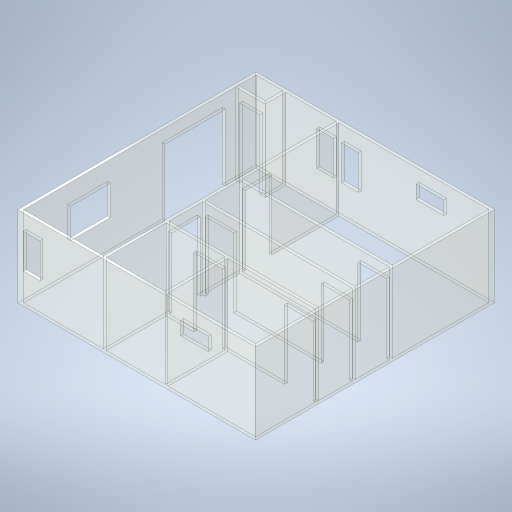
# Autodesk Inventor part: Interior_Walls
Saved by Autodesk Inventor 2024 (Build 280153000, 153)
## iProperties
Created: 2023-05-16
Part Number: Interior_Walls
Material: Steel
Document SubType Name: Modeling
Designer: Tom
Density: 7.85 g/cm^3
Appearance: Clear
Mass: 7.46669e+07 g
Surface Area: 2.27384e+06 cm^2
Volume: 9.51171e+06 cm^3
Author: Tom
Autodesk Inventor part; units mm, degrees
ref_plane "YZ Plane" through (0, 0, 0) normal (1, 0, 0) x (0, 1, 0)
ref_plane "XZ Plane" through (0, 0, 0) normal (0, 1, 0) x (-1, 0, 0)
ref_plane "XY Plane" through (0, 0, 0) normal (0, 0, 1) x (1, 0, 0)
sketch "Sketch1" plane through (0, 0, 0) normal (0, 1, 0) x (-1, 0, 0)
  line L0 (3606.8, -3606.8) -> (-3606.8, -3606.8)
  line L1 (-3606.8, -3606.8) -> (-3594.1, 3606.8)
  line L2 (-3594.1, 3606.8) -> (3594.1, 3606.8)
  line L3 (3594.1, 3606.8) -> (3606.8, -3606.8)
  line L4 (0, -3606.8) -> (0, 3606.8)
  line L5 (3600.45, 0) -> (-3600.45, 0)
  line L6 (3505.3564, 3517.9) -> (-3505.3564, 3517.9)
  line L7 (-3505.3564, 3517.9) -> (-3517.7433, -3517.9)
  line L8 (-3517.7433, -3517.9) -> (3517.7433, -3517.9)
  line L9 (3517.7433, -3517.9) -> (3505.3564, 3517.9)
  line L10 (-2204.4316, 514.35) -> (-2204.4316, 603.25)
  line L11 (5.3684, -603.25) -> (5.3684, -514.35)
  point P0 (0, 0)
  point P1 (0, 0)
  point P2 (-3511.5499, 0)
  dimension "d1" = 7213.6
  dimension "d2" = 12.7
  dimension "d4" = 7188.2
  dimension "d5" = 7213.6
  dimension "d6" = 88.9
  constraints: 24 end point, 6 midpoint, 2 parallel, 1 coincident, 1 horizontal, 1 perpendicular, 3 other
  measures "d1" distance of L0.start L0.end
  measures "d2" horizontal distance of L0.start L2.end
  measures "d4" distance of L1.end L2.end
  measures "d5" distance of L0.end L1.end
  measures "d6" distance between parallel lines of L2 L6
extrude "Extrusion1" add sketch "Sketch1" along normal blind 2438.4 contours L0 L4 L8 L9 L5 L3 | L0 L1 L5 L7 L8 L4 | L5 L9 L6 L4 L2 L3 | L1 L2 L4 L6 L7 L5
sketch "Sketch2" plane through (0, 2438.4, 0) normal (0, 1, 0) x (1, 0, 0)
  line L0 (-3517.7433, 3517.9) -> (3517.7433, 3517.9) projected
  line L1 (3505.3564, -3517.9) -> (-3505.3564, -3517.9) projected
  line L2 (-3517.7433, 3517.9) -> (3517.7433, 3517.9) projected
  line L3 (3505.3564, -3517.9) -> (-3505.3564, -3517.9) projected
  line L4 (3517.7433, 3517.9) -> (3505.3564, -3517.9) projected
  line L5 (-1009.4936, -1619.25) -> (3508.5426, -1619.25)
  line L6 (3508.5426, -1619.25) -> (3508.5426, -1708.15)
  line L7 (3508.5426, -1708.15) -> (-1009.4936, -1708.15)
  line L8 (857.4064, -1708.15) -> (768.5064, -1708.15)
  line L9 (768.5064, -1708.15) -> (768.5064, -3517.9)
  line L10 (768.5064, -3517.9) -> (857.4064, -3517.9)
  line L11 (857.4064, -3517.9) -> (857.4064, -1708.15)
  line L12 (-1009.4936, -3517.9) -> (-1009.4936, 3517.9)
  line L13 (-1098.3936, 3517.9) -> (-1098.3936, -3517.9)
  line L14 (-1009.4936, 3517.9) -> (-1098.3936, 3517.9)
  line L15 (-1009.4936, -3517.9) -> (-1098.3936, -3517.9)
  line L16 (-5.3684, -603.25) -> (2204.4316, -603.25) projected
  line L17 (-1009.4936, -603.25) -> (-1009.4936, -514.35)
  line L18 (-3505.3564, -3517.9) -> (-3517.7433, 3517.9) projected
  line L19 (-3516.6477, 2895.6) -> (-2614.9477, 2895.6)
  line L20 (-2703.8477, 2984.5) -> (-3516.6477, 2984.5)
  line L21 (-3516.6477, 2984.5) -> (-3516.6477, 2895.6)
  line L22 (-2703.8477, 2984.5) -> (-2703.8477, 3517.9)
  line L23 (-2703.8477, 3517.9) -> (-2614.9477, 3517.9)
  line L24 (-2614.9477, 3517.9) -> (-2614.9477, 2895.6)
  line L25 (-1009.4936, -603.25) -> (3510.6443, -603.25)
  line L26 (3510.6443, -603.25) -> (3510.6443, -514.35)
  line L27 (3510.6443, -514.35) -> (-1009.4936, -514.35)
  line L28 (-1009.4936, -514.35) -> (-1009.4936, -603.25)
  line L29 (-1009.4936, -1708.15) -> (-1009.4936, -1619.25)
  line L30 (-1009.4936, 514.35) -> (3512.6119, 514.35)
  line L31 (3512.6119, 514.35) -> (3512.6119, 603.25)
  line L32 (3512.6119, 603.25) -> (-1009.4936, 603.25)
  line L33 (-1009.4936, 603.25) -> (-1009.4936, 514.35)
  point P0 (0, 0)
  point P1 (857.4064, -3517.9)
  point P2 (768.5064, -1708.15)
  point P3 (-1098.3936, 3517.9)
  point P4 (-1098.3936, -3517.9)
  point P5 (-1009.4936, -3517.9)
  point P6 (-2614.9477, 3517.9)
  point P7 (-2703.8477, 3517.9)
  point P8 (-1009.4936, 603.25)
  dimension "d41" = 88.9
  dimension "d44" = 2647.95
  dimension "d45" = 1778
  dimension "d88" = 533.4
  dimension "d90" = 812.8
  dimension "d137" = 1016
  dimension "d138" = 514.35
  dimension "d139" = 514.35
  constraints: 54 end point, 16 point on line, 10 parallel, 9 perpendicular, 7 equal length, 5 horizontal, 2 collinear
  measures "d41" distance between parallel lines of L13 L12
  measures "d44" distance from line of L1.start L11
  measures "d45" distance between parallel lines of L9 L12
  measures "d88" distance of L20.start L22.end
  measures "d90" distance of L20.start L20.end
  measures "d137" distance between parallel lines of L5 L25
  measures "d138" distance from line of point (0, 0) L27
  measures "d139" distance from line of L30 point (0, 0)
extrude "Extrusion2" add sketch "Sketch2" against normal blind 2438.4 contours L0 L24 L19 L21 L20 L22 | L0 L12 L1 L13 | L32 L4 L30 L12 | L9 L7 L11 L1 | L12 L5 L6 L7 | L31 L30 L4 | L27 L4 L25 L16 L12 | L26 L25 L4
sketch "Sketch3" plane through (768.5064, 2438.4, 1708.15) normal (0, 0, 1) x (1, 0, 0)
  line L0 (-1778, -2438.4) -> (2740.0362, -2438.4) projected
  line L1 (2663.8362, -2438.4) -> (1800.2362, -2438.4)
  line L2 (1800.2362, -2438.4) -> (1800.2362, -355.6)
  line L3 (1800.2362, -355.6) -> (2663.8362, -355.6)
  line L4 (2663.8362, -355.6) -> (2663.8362, -2438.4)
  line L5 (2740.0362, 0) -> (2740.0362, -2438.4) projected
  point P0 (-768.5064, -2438.4)
  point P1 (-1526.4792, -2438.4)
  dimension "d36" = 76.2
  dimension "d37" = 863.6
  dimension "d38" = 2082.8
  constraints: 8 end point, 2 parallel, 1 horizontal, 1 perpendicular, 1 point on line
  measures "d36" distance between parallel lines of L5 L4
  measures "d37" distance of L2.end L3.end
  measures "d38" distance of L1.end L2.end
extrude "Extrusion3" cut sketch "Sketch3" against normal up to surface (2311.4 mm away)
ref_plane "Work Plane1" through (3038.6426, 2082.8, 1708.15) normal (0, -1, 0) x (1, 0, 0)
sketch "Sketch4" plane through (-0.1006, 2082.8, 57.15) normal (0, 1, 0) x (1, 0, 0)
  line L0 (857.507, -1651) -> (3508.6432, -1651) projected
  arc A0 (2594.2432, -1651) -> (3400.6932, -2457.45) centre (3400.6932, -1651) ccw
  line L1 (3400.6932, -1651) -> (2594.2432, -1651)
  line L2 (3400.6932, -1651) -> (3400.6932, -2457.45)
  point P0 (0.1006, 57.15)
  point P1 (3432.4432, -1651)
  dimension "d46" = 31.75
  dimension "d48" = 806.45
  constraints: 4 end point, 2 point on circle, 2 point on line, 1 centre point, 1 coincident, 1 perpendicular
  measures "d46" distance of point (3432.443, -1651) point (3400.693, -1651)
  measures "d48" distance of L1.start L1.end
sketch "Sketch5" plane through (-3594.1, 0, 3606.8) normal (0, 0, 1) x (1, 0, 0)
  line L0 (4927.6, 2006.6) -> (5753.1, 2006.6)
  line L1 (5753.1, 2006.6) -> (5753.1, 1600.2)
  line L2 (5753.1, 1600.2) -> (4927.6, 1600.2)
  line L3 (4927.6, 1600.2) -> (4927.6, 2006.6)
  line L4 (0, 0) -> (7188.2, 0) projected
  line L5 (7200.9, 0) -> (7200.9, 2438.4) projected
  point P0 (3594.1, 0)
  dimension "d51" = 2006.6
  dimension "d53" = 825.5
  dimension "d54" = 406.4
  dimension "d165" = 1447.8
  constraints: 8 end point, 2 parallel, 1 horizontal, 1 perpendicular
  measures "d51" distance between parallel lines of L4 L0
  measures "d53" distance of L0.start L0.end
  measures "d54" distance between parallel lines of L2 L0
  measures "d165" distance between parallel lines of L5 L1
extrude "Extrusion4" cut sketch "Sketch5" against normal up to surface (88.9 mm away)
sketch "Sketch6" plane through (3606.8, 0, -3606.8) normal (0, 0, -1) x (-1, 0, 0)
  line L0 (1447.8, 2006.6) -> (2286, 2006.6)
  line L1 (2286, 2006.6) -> (2286, 1600.2)
  line L2 (2286, 1600.2) -> (1447.8, 1600.2)
  line L3 (1447.8, 1600.2) -> (1447.8, 2006.6)
  line L4 (0, 0) -> (7213.6, 0) projected
  line L5 (0, 0) -> (0, 2438.4) projected
  point P0 (3606.8, 0)
  point P1 (1447.8, 1803.4)
  dimension "d57" = 2006.6
  dimension "d58" = 406.4
  dimension "d59" = 838.2
  dimension "d60" = 1447.8
  constraints: 8 end point, 2 parallel, 1 horizontal, 1 midpoint, 1 perpendicular
  measures "d57" distance between parallel lines of L4 L0
  measures "d58" distance of L2.end L0.start
  measures "d59" distance of L1.end L2.end
  measures "d60" distance from line of L5 point (1447.8, 1803.4)
extrude "Extrusion5" cut sketch "Sketch6" against normal up to surface (88.9 mm away)
sketch "Sketch7" plane through (-3517.7433, 0, -3517.9) normal (0.9999985, 0, -0.0017606) x (-0.0017606, 0, -0.9999985)
  line L0 (-927.1, 0) -> (-2755.9, 0)
  line L1 (-2755.9, 0) -> (-2755.9, 2006.6)
  line L2 (-2755.9, 2006.6) -> (-927.1, 2006.6)
  line L3 (-927.1, 2006.6) -> (-927.1, 0)
  line L4 (0, 0) -> (0, 2438.4) projected
  line L5 (-7035.8109, 0) -> (-622.301, 0) projected
  point P0 (-3524.0877, 0)
  dimension "d63" = 927.1
  dimension "d64" = 2006.6
  dimension "d65" = 1828.8
  constraints: 8 end point, 2 parallel, 1 collinear, 1 horizontal, 1 perpendicular
  measures "d63" distance between parallel lines of L3 L4
  measures "d64" distance of L0.end L1.end
  measures "d65" distance of L1.end L2.end
extrude "Extrusion6" cut sketch "Sketch7" against normal up to surface (88.9 mm away)
sketch "Sketch8" plane through (-3594.1, 0, 3606.8) normal (-0.9999985, 0, 0.0017606) x (0.0017606, 0, 0.9999985)
  line L0 (-2717.8, 1816.1) -> (-1511.3, 1816.1)
  line L1 (-1511.3, 1816.1) -> (-1511.3, 914.4)
  line L2 (-1511.3, 914.4) -> (-2717.8, 914.4)
  line L3 (-2717.8, 914.4) -> (-2717.8, 1816.1)
  line L4 (0, 0) -> (0, 2438.4) projected
  line L5 (-7213.6112, 0) -> (0, 0) projected
  point P0 (-3600.4668, 0)
  point P1 (-4368.6545, 0)
  dimension "d71" = 2717.8
  dimension "d72" = 901.7
  dimension "d73" = 1206.5
  dimension "d111" = 914.4
  constraints: 8 end point, 2 parallel, 1 horizontal, 1 perpendicular
  measures "d71" distance between parallel lines of L3 L4
  measures "d72" distance of L0.end L1.end
  measures "d73" distance of L1.end L2.end
  measures "d111" distance from line of L5 L2.end
extrude "Extrusion7" cut sketch "Sketch8" against normal up to surface (88.9 mm away)
sketch "Sketch9" plane through (3517.7433, 0, -3517.9) normal (0, 0, 1) x (1, 0, 0)
  line L0 (-4451.037, 1955.8) -> (-3943.037, 1955.8)
  line L1 (-3943.037, 1955.8) -> (-3943.037, 914.4)
  line L2 (-3943.037, 914.4) -> (-4451.037, 914.4)
  line L3 (-4451.037, 914.4) -> (-4451.037, 1955.8)
  line L4 (-7035.4867, 0) -> (0, 0) projected
  line L5 (-4527.237, 2438.4) -> (-4527.237, 0) projected
  point P0 (-3517.7433, 0)
  dimension "d76" = 1041.4
  dimension "d77" = 914.4
  dimension "d78" = 76.2
  dimension "d79" = 508
  constraints: 8 end point, 2 parallel, 1 horizontal, 1 perpendicular
  measures "d76" distance of L0.end L1.end
  measures "d77" distance between parallel lines of L4 L2
  measures "d78" distance between parallel lines of L5 L3
  measures "d79" distance of L0.start L0.end
extrude "Extrusion8" cut sketch "Sketch9" against normal up to surface (88.9 mm away)
sketch "Sketch10" plane through (-3517.7433, 0, -3517.9) normal (0, 0, 1) x (1, 0, 0)
  line L0 (2343.1497, 914.4) -> (1835.1497, 914.4)
  line L1 (1835.1497, 914.4) -> (1835.1497, 1955.8)
  line L2 (1835.1497, 1955.8) -> (2343.1497, 1955.8)
  line L3 (2343.1497, 1955.8) -> (2343.1497, 914.4)
  line L4 (2419.3497, 0) -> (2419.3497, 2438.4) projected
  line L5 (0, 0) -> (7035.4867, 0) projected
  point P0 (3517.7433, 0)
  dimension "d82" = 76.2
  dimension "d83" = 914.4
  dimension "d84" = 508
  dimension "d85" = 1041.4
  constraints: 8 end point, 2 parallel, 1 horizontal, 1 perpendicular
  measures "d82" distance between parallel lines of L4 L3
  measures "d83" distance between parallel lines of L5 L0
  measures "d84" distance of L1.end L2.end
  measures "d85" distance of L0.end L1.end
extrude "Extrusion9" cut sketch "Sketch10" against normal up to surface (88.9 mm away)
sketch "Sketch11" plane through (-3516.6477, 2438.4, -2895.6) normal (0, 0, 1) x (1, 0, 0)
  line L0 (0, -2438.4) -> (812.8, -2438.4) projected
  line L1 (736.6, -2438.4) -> (127, -2438.4)
  line L2 (127, -2438.4) -> (127, -355.6)
  line L3 (127, -355.6) -> (736.6, -355.6)
  line L4 (736.6, -355.6) -> (736.6, -2438.4)
  line L5 (901.7, 0) -> (901.7, -2438.4) projected
  point P0 (3516.6477, -2438.4)
  dimension "d91" = 165.1
  dimension "d92" = 609.6
  dimension "d95" = 2082.8
  constraints: 8 end point, 2 parallel, 1 horizontal, 1 perpendicular, 1 point on line
  measures "d91" distance between parallel lines of L5 L4
  measures "d92" distance of L2.end L3.end
  measures "d95" distance of L1.end L2.end
extrude "Extrusion10" cut sketch "Sketch11" against normal up to surface (88.9 mm away)
sketch "Sketch12" plane through (-1009.4936, 2438.4, 1708.15) normal (0, 0, 1) x (1, 0, 0)
  line L0 (1778, -2438.4) -> (0, -2438.4) projected
  line L1 (1701.8, -2438.4) -> (838.2, -2438.4)
  line L2 (838.2, -2438.4) -> (838.2, -355.6)
  line L3 (838.2, -355.6) -> (1701.8, -355.6)
  line L4 (1701.8, -355.6) -> (1701.8, -2438.4)
  line L5 (1778, 0) -> (1778, -2438.4) projected
  point P0 (1009.4936, -2438.4)
  dimension "d96" = 76.2
  dimension "d97" = 863.6
  dimension "d98" = 2082.8
  constraints: 8 end point, 2 parallel, 1 horizontal, 1 perpendicular, 1 point on line
  measures "d96" distance between parallel lines of L5 L4
  measures "d97" distance of L2.end L3.end
  measures "d98" distance of L1.end L2.end
extrude "Extrusion11" cut sketch "Sketch12" against normal up to surface (88.9 mm away)
sketch "Sketch15" plane through (-3594.1, 0, 3606.8) normal (0, 0, 1) x (1, 0, 0)
  line L0 (164.9436, 1955.8) -> (672.9436, 1955.8)
  line L1 (672.9436, 1955.8) -> (672.9436, 914.4)
  line L2 (672.9436, 914.4) -> (164.9436, 914.4)
  line L3 (164.9436, 914.4) -> (164.9436, 1955.8)
  line L4 (0, 0) -> (7188.2, 0) projected
  point P0 (3594.1, 0)
  point P1 (88.7436, 2438.4)
  dimension "d113" = 1041.4
  dimension "d114" = 508
  dimension "d115" = 76.2
  dimension "d116" = 914.4
  constraints: 8 end point, 2 parallel, 1 horizontal, 1 perpendicular
  measures "d113" distance of L0.end L1.end
  measures "d114" distance of L0.start L0.end
  measures "d115" distance from line of L3 point (88.744, 2438.4)
  measures "d116" distance between parallel lines of L4 L2
extrude "Extrusion14" cut sketch "Sketch15" against normal up to surface (88.9 mm away)
sketch "Sketch16" plane through (-1098.3936, 2438.4, -3517.9) normal (-1, 0, 0) x (0, 0, 1)
  line L0 (5137.15, 0) -> (5137.15, -2438.4) projected
  line L1 (4121.15, 0) -> (4121.15, -2438.4) projected
  line L2 (7035.8, -2438.4) -> (0, -2438.4) projected
  line L3 (5060.95, -2438.4) -> (4197.35, -2438.4)
  line L4 (4197.35, -2438.4) -> (4197.35, -355.6)
  line L5 (4197.35, -355.6) -> (5060.95, -355.6)
  line L6 (5060.95, -355.6) -> (5060.95, -2438.4)
  point P0 (3517.9, -2438.4)
  point P1 (7035.8, -2470.15)
  point P2 (0, -2470.15)
  point P3 (0, -2438.4)
  dimension "d122" = 76.2
  dimension "d123" = 863.6
  dimension "d124" = 2082.8
  constraints: 8 end point, 2 parallel, 1 horizontal, 1 perpendicular, 2 other
  measures "d122" distance between parallel lines of L0 L6
  measures "d123" distance of L4.end L5.end
  measures "d124" distance of L3.end L4.end
extrude "Extrusion15" cut sketch "Sketch16" against normal up to surface (88.9 mm away)
sketch "Sketch22" plane through (-1009.4936, 2438.4, -603.25) normal (1, 0, 0) x (0, 0, -1)
  line L0 (2914.65, -2438.4) -> (0, -2438.4) projected
  line L1 (76.2, -2438.4) -> (889, -2438.4)
  line L2 (889, -2438.4) -> (889, -355.6)
  line L3 (889, -355.6) -> (76.2, -355.6)
  line L4 (76.2, -355.6) -> (76.2, -2438.4)
  point P0 (-603.25, -2438.4)
  point P1 (0, 0)
  dimension "d155" = 76.2
  dimension "d156" = 812.8
  dimension "d157" = 2082.8
  constraints: 8 end point, 2 parallel, 1 horizontal, 1 perpendicular, 1 point on line
  measures "d155" distance from line of point (0, 0) L4
  measures "d156" distance of L2.end L3.end
  measures "d157" distance of L1.end L2.end
extrude "Extrusion21" cut sketch "Sketch22" against normal up to surface (88.9 mm away)
sketch "Sketch23" plane through (-1009.4936, 2438.4, 603.25) normal (0, 0, 1) x (1, 0, 0)
  line L0 (3578.2362, -2438.4) -> (0, -2438.4) projected
  line L1 (76.2, -2438.4) -> (939.8, -2438.4)
  line L2 (939.8, -2438.4) -> (939.8, -355.6)
  line L3 (939.8, -355.6) -> (76.2, -355.6)
  line L4 (76.2, -355.6) -> (76.2, -2438.4)
  point P0 (1009.4936, -2438.4)
  point P1 (0, 0)
  point P2 (939.8, -2438.4)
  dimension "d160" = 76.2
  dimension "d161" = 2082.8
  dimension "d162" = 863.6
  constraints: 8 end point, 2 parallel, 1 horizontal, 1 perpendicular, 1 point on line
  measures "d160" distance from line of point (0, 0) L4
  measures "d161" distance of L1.end L2.end
  measures "d162" distance of L2.end L3.end
extrude "Extrusion22" cut sketch "Sketch23" against normal up to surface (88.9 mm away)
body "Solid1"
